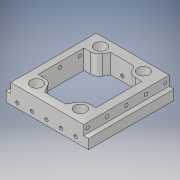
# Autodesk Inventor part: Крышка
Saved by Autodesk Inventor 2019 (Build 230136000, 136)
## iProperties
Created: 2021-03-11
Part Number: Крышка
Material: Iron, Malleable
Document SubType Name: Modeling
Designer: Ivan
Density: 7.15 g/cm^3
Appearance: Aluminum - Dark
Author: Ivan
Autodesk Inventor part; units mm, degrees
ref_plane "YZ Plane" through (0, 0, 0) normal (1, 0, 0) x (0, 1, 0)
ref_plane "XZ Plane" through (0, 0, 0) normal (0, 1, 0) x (-1, 0, 0)
ref_plane "XY Plane" through (0, 0, 0) normal (0, 0, 1) x (1, 0, 0)
sketch "Эскиз1" plane through (0, 0, 0) normal (0, 1, 0) x (-1, 0, 0)
  line L0 (0, -34.7034) -> (-12.0112, -34.7034)
  line L1 (-12.0112, -34.7034) -> (-15.1483, -29.3519)
  arc A0 (-15.1483, -29.3519) -> (-22.9532, -24.8801) centre (-22.9532, -33.9273) ccw
  line L2 (-22.9532, -24.8801) -> (-29.7721, -24.8801)
  line L3 (-29.7721, -24.8801) -> (-29.7721, -9.7931)
  line L4 (-29.7721, -9.7931) -> (-32.9968, -4.2922)
  arc A1 (-33.0385, 4.7866) -> (-32.9968, -4.2922) centre (-25.1918, 0.2831) ccw
  line L5 (-33.0385, 4.7866) -> (-31.4302, 7.5887)
  line L6 (-31.4302, 7.5887) -> (-31.4302, 22.3943)
  line L7 (-31.4302, 22.3943) -> (-23.0086, 22.3943)
  arc A2 (-23.0086, 22.3943) -> (-15.1619, 26.938) centre (-23.0086, 31.4415) ccw
  line L8 (-15.1619, 26.938) -> (-10.7051, 34.7034)
  line L9 (-10.7051, 34.7034) -> (0, 34.7034)
  line L10 (-43.3228, -44.5266) -> (41.6772, -44.5266)
  line L11 (41.6772, -44.5266) -> (41.6772, 43.4734)
  line L12 (41.6772, 43.4734) -> (-43.3228, 43.4734)
  line L13 (-43.3228, 43.4734) -> (-43.3228, -44.5266)
  circle A3 centre (-22.653, 31.1943) radius 3.6264
  circle A4 centre (22.5749, 31.1943) radius 3.509
  circle A5 centre (22.5749, -34.7034) radius 3.2033
  circle A6 centre (-21.6298, -34.7034) radius 3.1306
  line L14 (0, 34.7034) -> (0, -34.7034)
  line L15 (0, -34.7034) -> (12.0112, -34.7034)
  line L16 (12.0112, -34.7034) -> (15.1483, -29.3519)
  arc A7 (22.9532, -24.8801) -> (15.1483, -29.3519) centre (22.9532, -33.9273) ccw
  line L17 (22.9532, -24.8801) -> (29.7721, -24.8801)
  line L18 (29.7721, -24.8801) -> (29.7721, -9.7931)
  line L19 (29.7721, -9.7931) -> (32.9968, -4.2922)
  arc A8 (32.9968, -4.2922) -> (33.0385, 4.7866) centre (25.1918, 0.2831) ccw
  line L20 (33.0385, 4.7866) -> (31.4302, 7.5887)
  line L21 (31.4302, 7.5887) -> (31.4302, 22.3943)
  line L22 (31.4302, 22.3943) -> (23.0086, 22.3943)
  arc A9 (15.1619, 26.938) -> (23.0086, 22.3943) centre (23.0086, 31.4415) ccw
  line L23 (15.1619, 26.938) -> (10.7051, 34.7034)
  line L24 (10.7051, 34.7034) -> (0, 34.7034)
  line L25 (0, 34.7034) -> (10.7051, 34.7034)
  point P0 (-146.6453, 374.7827)
  point P1 (0, 0)
  dimension "d15" = 88
  dimension "d16" = 85
  constraints: 52 end point, 27 symmetric about line, 12 point on circle, 10 centre point, 1 horizontal, 1 midpoint, 3 other
  measures "d15" distance between parallel lines of L10 L12
  measures "d16" distance between parallel lines of L13 L11
extrude "Выдавливание1" add sketch "Эскиз1" along normal blind 10
sketch "Sketch3" plane through (0, 10, 0) normal (0, 1, 0) x (1, 0, 0)
  line L0 (-31.4302, -7.5887) -> (-31.4302, -22.3943) projected
  line L1 (-29.7721, 9.7931) -> (-32.9968, 4.2922) projected
  line L2 (33.0385, -4.7866) -> (31.4302, -7.5887) projected
  line L3 (31.4302, -7.5887) -> (31.4302, 6.9645)
  line L4 (32.9968, 4.2922) -> (29.7721, 9.7931) projected
  line L5 (-31.4302, -7.5887) -> (-33.0385, -4.7866) projected
  line L6 (-31.4302, -7.5887) -> (-31.4302, 6.9645)
  arc A0 (-32.9968, 4.2922) -> (-33.0385, -4.7866) centre (-25.1918, -0.2831) ccw projected
  arc A1 (33.0385, -4.7866) -> (32.9968, 4.2922) centre (25.1918, -0.2831) ccw projected
  line L7 (29.7721, 24.8801) -> (29.7721, 9.7931) projected
  line L8 (-29.7721, 24.8801) -> (-29.7721, 9.7931) projected
  line L9 (-29.7721, 24.8801) -> (-29.7721, -22.3943)
  line L10 (-23.0086, -22.3943) -> (-31.4302, -22.3943) projected
  line L11 (29.7721, 9.7931) -> (29.7721, 24.8801) projected
  line L12 (29.7721, 24.8801) -> (29.7721, -22.3943)
  line L13 (31.4302, -22.3943) -> (23.0086, -22.3943) projected
  line L14 (31.4302, -7.5887) -> (31.4302, -22.3943) projected
  point P0 (0, 0)
  constraints: 8 end point, 8 point on line, 2 collinear, 1 parallel, 1 vertical
extrude "Extrusion2" add sketch "Sketch3" against normal up to surface (10 mm away)
sketch "Sketch4" plane through (0, 10, 0) normal (0, 1, 0) x (1, 0, 0)
  line L0 (43.3228, 44.5266) -> (-41.6772, 44.5266) projected
  line L1 (-36.6772, 44.5266) -> (-36.6772, -43.4734)
  line L2 (-41.6772, -43.4734) -> (43.3228, -43.4734) projected
  line L3 (38.3228, 44.5266) -> (38.3228, -43.4734)
  line L4 (-22.9532, 24.8801) -> (-29.7721, 24.8801) projected
  line L5 (-29.7721, 24.8801) -> (-29.7721, 44.5266)
  line L6 (-29.7721, -22.3943) -> (-23.0086, -22.3943) projected
  line L7 (-29.7721, -22.3943) -> (-29.7721, -43.4734)
  line L8 (-31.4302, -22.3943) -> (-31.4302, 6.9645) projected
  line L9 (-31.4302, 6.9645) -> (-29.7721, 9.7931) projected
  line L10 (-29.7721, -22.3943) -> (-29.7721, 24.8801) projected
  line L11 (29.7721, 24.8801) -> (29.7721, -22.3943) projected
  line L12 (29.7721, 9.7931) -> (31.4302, 6.9645) projected
  line L13 (31.4302, 6.9645) -> (31.4302, -22.3943) projected
  line L14 (29.7721, -22.3943) -> (23.0086, -22.3943) projected
  line L15 (29.7721, 24.8801) -> (22.9532, 24.8801) projected
  line L16 (29.7721, 24.8801) -> (29.7721, 44.5266)
  line L17 (29.7721, -22.3943) -> (29.7721, -43.4734)
  line L18 (-41.6772, 44.5266) -> (-41.6772, -43.4734) projected
  line L19 (-41.6772, -43.4734) -> (43.3228, -43.4734) projected
  line L20 (43.3228, -43.4734) -> (43.3228, 44.5266) projected
  line L21 (43.3228, 44.5266) -> (-41.6772, 44.5266) projected
  circle A0 centre (21.6298, 34.7034) radius 3.1306 projected
  circle A1 centre (-22.5749, 34.7034) radius 3.2033 projected
  circle A2 centre (-22.5749, -31.1943) radius 3.509 projected
  circle A3 centre (22.653, -31.1943) radius 3.6264 projected
  line L22 (-12.0112, 34.7034) -> (12.0112, 34.7034) projected
  line L23 (12.0112, 34.7034) -> (15.1483, 29.3519) projected
  arc A4 (15.1483, 29.3519) -> (22.9532, 24.8801) centre (22.9532, 33.9273) ccw projected
  line L24 (22.9532, 24.8801) -> (29.7721, 24.8801) projected
  line L25 (29.7721, 24.8801) -> (29.7721, -22.3943) projected
  line L26 (29.7721, -22.3943) -> (23.0086, -22.3943) projected
  arc A5 (23.0086, -22.3943) -> (15.1619, -26.938) centre (23.0086, -31.4415) ccw projected
  line L27 (15.1619, -26.938) -> (10.7051, -34.7034) projected
  line L28 (10.7051, -34.7034) -> (-10.7051, -34.7034) projected
  line L29 (-10.7051, -34.7034) -> (-15.1619, -26.938) projected
  arc A6 (-15.1619, -26.938) -> (-23.0086, -22.3943) centre (-23.0086, -31.4415) ccw projected
  line L30 (-23.0086, -22.3943) -> (-29.7721, -22.3943) projected
  line L31 (-29.7721, -22.3943) -> (-29.7721, 24.8801) projected
  line L32 (-29.7721, 24.8801) -> (-22.9532, 24.8801) projected
  arc A7 (-22.9532, 24.8801) -> (-15.1483, 29.3519) centre (-22.9532, 33.9273) ccw projected
  line L33 (-15.1483, 29.3519) -> (-12.0112, 34.7034) projected
  line L34 (43.3228, 44.5266) -> (-41.6772, 44.5266) projected
  point P0 (0, 0)
  dimension "d14" = 5
  dimension "d19" = 5
  constraints: 14 end point, 12 point on line, 2 perpendicular, 1 parallel, 1 vertical
  measures "d14" distance between parallel lines of L18 L1
  measures "d19" distance between parallel lines of L20 L3
extrude "Extrusion3" add sketch "Sketch4" along normal blind 10 contours L3 L2 L17 L11 L16 L0 | L16 L15 A4 L23 L22 L33 A7 L4 L5 L0 | L5 L10 L7 L2 L1 L0 | L2 L7 L6 A6 L29 L28 L27 A5 L14 L17
sketch "Sketch5" plane through (0, 20, 0) normal (0, 1, 0) x (1, 0, 0)
  circle A0 centre (22.653, -31.1943) radius 3.6264 projected
  circle A1 centre (22.653, -31.1943) radius 6
  point P0 (0, 0)
  dimension "d11" = 12
  constraints: 1 centre point, 1 coincident
  measures "d11" diameter of A1
extrude "Extrusion4" cut sketch "Sketch5" against normal blind 15 contours A0 | A1
sketch "Sketch6" plane through (0, 20, 0) normal (0, 1, 0) x (1, 0, 0)
  circle A0 centre (-22.5749, -31.1943) radius 3.509 projected
  circle A1 centre (-22.5749, 34.7034) radius 3.2033 projected
  circle A2 centre (21.6298, 34.7034) radius 3.1306 projected
  circle A3 centre (-22.5749, 34.7034) radius 3.2033 projected
  point P0 (0, 0)
  constraints: 3 coincident
pattern_sketch "Sketch Driven Pattern1" of "Extrusion4" from (22.653, 20, 31.1943) copies at (-22.5749, 20, 31.1943) at (-22.5749, 20, -34.7034) at (21.6298, 20, -34.7034)
sketch "Sketch7" plane through (38.3228, 10, 43.4734) normal (1, 0, 0) x (0, 0, -1)
  circle A0 centre (4, 5) radius 1.75
  line L0 (0, 0) -> (88, 0) projected
  line L1 (0, 0) -> (0, 10) projected
  point P0 (43.4734, -10)
  dimension "d20" = 3.5
  dimension "d21" = 5
  dimension "d22" = 4
  constraints: 1 centre point
  measures "d20" diameter of A0
  measures "d21" distance from line of L0 A0.centre
  measures "d22" distance from line of L1 A0.centre
hole "Hole1" at (38.3228, 15, 39.4734) direction (-1, 0, 0) diameter 3.5 depth 10 tip angle 120
sketch "Sketch8" plane through (-41.6772, 0, 43.4734) normal (0, 0, 1) x (1, 0, 0)
  circle A0 centre (41.6772, 5) radius 1.75
  point P0 (41.6772, 0)
  dimension "d28" = 3.5
  dimension "d29" = 5
  constraints: 1 centre point, 1 vertical alignment
  measures "d28" diameter of A0
  measures "d29" distance of point (41.677, 0) A0.centre
thread "Thread9" size "M3.5x0.6" class "6H" standard "ANSI Metric M Profile" full length
pattern_linear "Rectangular Pattern3" count 5 spacing 20 along (0, 0, -1) of "Hole1"
thread "Thread5" size "M8x1.25" class "6H" standard "ANSI Metric M Profile" full length
thread "Thread6" size "M7x1" class "6H" standard "ANSI Metric M Profile" full length
thread "Thread7" size "M7x1" class "6H" standard "ANSI Metric M Profile" full length
thread "Thread8" size "M8x1.25" class "6H" standard "ANSI Metric M Profile" full length
mirror "Mirror3" about plane through (0, 0, 0) normal (1, 0, 0) of "Hole1", "Rectangular Pattern3"
hole "Hole2" at (0, 5, 43.4734) direction (0, 0, -1) diameter 3.5 depth 10 tip angle 120
thread "Thread10" size "M3.5x0.6" class "6H" standard "ANSI Metric M Profile" full length
pattern_linear "Rectangular Pattern4" count 5 spacing 15 along (1, 0, 0) of "Hole2" first direction both ways yes
ref_plane "Work Plane1" through (-36.6772, 20, -0.5266) normal (0, 0, -1) x (-1, 0, 0)
mirror "Mirror5" about plane through (-36.6772, 20, -0.5266) normal (0, 0, -1) of "Hole2", "Rectangular Pattern4"
equation "\"d19\" = d14"
